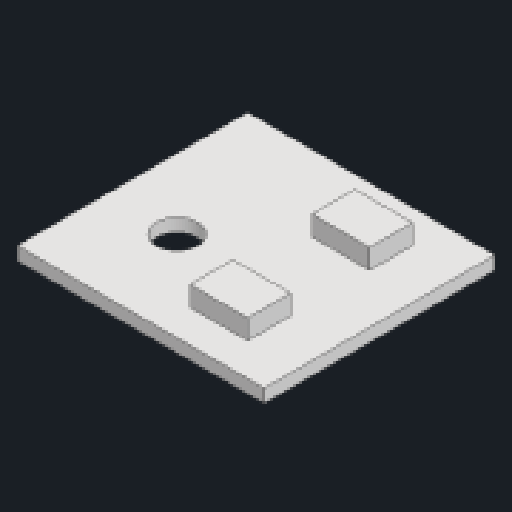
# Autodesk Inventor part: line_sensor
Saved by Autodesk Inventor 2023 (Build 270158000, 158)
## iProperties
Created: 2024-04-13
Part Number: line_sensor
Material: Generic
Document SubType Name: Modeling
Designer: szymo
Density: 1 g/cm^3
Appearance: Default
Author: szymo
Autodesk Inventor part; units mm, degrees
ref_plane "YZ Plane" through (0, 0, 0) normal (1, 0, 0) x (0, 1, 0)
ref_plane "XZ Plane" through (0, 0, 0) normal (0, 1, 0) x (-1, 0, 0)
ref_plane "XY Plane" through (0, 0, 0) normal (0, 0, 1) x (1, 0, 0)
sketch "Sketch1" plane through (0, 0, 0) normal (0, 1, 0) x (-1, 0, 0)
  line L0 (0, 0) -> (-15, 0)
  line L1 (-15, 0) -> (-15, -14)
  line L2 (-15, -14) -> (0, -14)
  line L3 (0, -14) -> (0, 0)
  line L4 (0, -4.2) -> (-15, -4.2)
  line L5 (-3, 0) -> (-3, -14)
  circle A0 centre (-4.25, -5.45) radius 1.25
  line L6 (-12, -2) -> (-14, -2)
  line L7 (-14, -2) -> (-14, -12)
  line L8 (-14, -12) -> (-12, -12)
  line L9 (-12, -12) -> (-12, -2)
  line L10 (-12, -2) -> (-8.5, -2)
  line L11 (-8.5, -2) -> (-8.5, -4.6)
  line L12 (-8.5, -4.6) -> (-12, -4.6)
  line L13 (-12, -4.6) -> (-12, -2)
  line L14 (-12, -12) -> (-8.5, -12)
  line L15 (-8.5, -12) -> (-8.5, -9.4)
  line L16 (-8.5, -9.4) -> (-12, -9.4)
  line L17 (-12, -9.4) -> (-12, -12)
  dimension "d0" = 15
  dimension "d1" = 14
  dimension "d2" = 4.2
  dimension "d3" = 3
  dimension "d4" = 2.5
  dimension "d5" = 10
  dimension "d6" = 2
  dimension "d7" = 2
  dimension "d8" = 2
  dimension "d9" = 1
  dimension "d10" = 3.5
  dimension "d11" = 3.5
  dimension "d12" = 2.6
  dimension "d13" = 2.6
  dimension "d14" = 2
  dimension "d15" = 2
  constraints: 36 end point, 8 parallel, 6 perpendicular, 6 point on line, 4 horizontal, 2 tangent, 1 centre point
  measures "d0" distance of L2.end L1.end
  measures "d1" distance of L1.end L0.end
  measures "d2" distance between parallel lines of L0 L4
  measures "d3" distance between parallel lines of L3 L5
  measures "d4" diameter of A0
  measures "d5" distance of L8.end L6.start
  measures "d6" distance of L7.end L8.end
  measures "d7" distance between parallel lines of L2 L8
  measures "d8" distance between parallel lines of L0 L6
  measures "d9" distance between parallel lines of L7 L1
  measures "d10" distance of L11.end L12.end
  measures "d11" distance of L16.end L15.end
  measures "d12" distance of L10.end L11.end
  measures "d13" distance of L14.end L15.end
  measures "d14" distance between parallel lines of L2 L14
  measures "d15" distance between parallel lines of L0 L10
extrude "Extrusion1" add sketch "Sketch1" against normal blind 0.8 contours L3 L4 L5 L0 | L5 L4 L11 L10 L6 L7 L1 L0 | L3 L2 L5 L4 | L5 A0 L4 | L4 L7 L8 L14 L15 L16 L9 L12 L11 A0 L5 L2 L1 | L7 L6 L9 L4 | L4 L9 L8 L7 | L11 L12 L9 L4 | L4 L9 L10 L11 | L9 L16 L15 L14
extrude "Extrusion2" add sketch "Sketch1" along normal blind 1.2 contours L11 L12 L9 L4 | L4 L9 L10 L11 | L9 L16 L15 L14
extrude "Extrusion3" add sketch "Sketch1" against normal blind 1.8 contours L7 L6 L9 L4 | L4 L9 L8 L7
equation "\"d7\" = d8"
body "Solid1"
